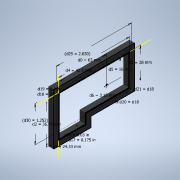
# Autodesk Inventor part: J010359
Saved by Autodesk Inventor 2020.3 (Build 243373000, 373)
## iProperties
RuleStatus: InUse
AfterDocSave0: file://Part Number Cleaner
Created: 2022-05-31
Part Number: J010359
Material: ACRYLIC, BLACK
Catalog Web Link: https://www.janelia.org/
Vendor: HHMI: JRC - jET
Document SubType Name: Modeling
Designer: arnoldj
Density: 1 g/cm^3
Appearance: Generic
Project: COMMON
Description: DOUT BASE PLATE
LAB/DEPT: COMMON
REQUESTING SCIENTIST: OCMMON
SURFACE ROUGHNESS: N/A
DESIGN DEPARTMENT: HHMI: JRC - jET
SPECIAL FINISH: NONE
ALTERED ITEM PART NUMBER: N/A
ALTERED ITEM VENDOR: N/A
ALTERED ITEM DESCRIPTION: N/A
Title: Standard
Author: arnoldj
Revision Number: 0
Autodesk Inventor part; units mm, degrees
ref_plane "YZ Plane" through (0, 0, 0) normal (1, 0, 0) x (0, 1, 0)
ref_plane "XZ Plane" through (0, 0, 0) normal (0, 1, 0) x (-1, 0, 0)
ref_plane "XY Plane" through (0, 0, 0) normal (0, 0, 1) x (1, 0, 0)
sketch "Sketch1" plane through (0, 0, 0) normal (1, 0, 0) x (0, 1, 0)
  line L0 (0, 18.823) -> (0, -81.823) projected
  line L1 (-50.323, 0) -> (13.573, 0) projected
  line L2 (0, 0) -> (0, -63)
  line L3 (0, -63) -> (-28, -63)
  line L4 (-28, -63) -> (-28, -24.33)
  line L5 (-28, -24.33) -> (-36.75, -24.33)
  line L6 (-36.75, -24.33) -> (-36.75, 0)
  line L7 (-36.75, 0) -> (0, 0)
  circle A0 centre (-16, -42.5) radius 1.575 construction
  line L8 (-35.988, -0.762) -> (-35.988, -23.568)
  line L9 (-35.988, -23.568) -> (-27.238, -23.568)
  line L10 (-27.238, -23.568) -> (-27.238, -62.238)
  line L11 (-27.238, -62.238) -> (-0.762, -62.238)
  line L12 (-0.762, -62.238) -> (-0.762, -0.762)
  line L13 (-0.762, -0.762) -> (-35.988, -0.762)
  line L14 (-41.195, 4.445) -> (-41.195, -28.775)
  line L15 (-41.195, -28.775) -> (-32.445, -28.775)
  line L16 (-32.445, -28.775) -> (-32.445, -67.445)
  line L17 (-32.445, -67.445) -> (4.445, -67.445)
  line L18 (4.445, -67.445) -> (4.445, 4.445)
  line L19 (4.445, 4.445) -> (-41.195, 4.445)
  line L20 (1.905, 1.905) -> (-29.905, 1.905) construction
  line L21 (-29.905, 1.905) -> (-29.905, -64.905) construction
  line L22 (-29.905, -64.905) -> (1.905, -64.905) construction
  line L23 (1.905, -64.905) -> (1.905, 1.905) construction
  dimension "d0" = 63
  dimension "d1" = 28
  dimension "d2" = 36.75
  dimension "d3" = 24.33
  dimension "d4" = 42.5
  dimension "d5" = 16
  dimension "d6" = 3.15
  dimension "d16" = 0.762
  dimension "d17" = 4.445
  dimension "d18" = 2.54
  dimension "d19" = 2.54
  dimension "d20" = 2.54
  dimension "d21" = 2.54
  dimension "d29" = 66.81
  dimension "d30" = 31.81
  constraints: 44 end point, 8 perpendicular, 3 horizontal, 2 coincident, 2 parallel, 2 point on line, 1 centre point, 10 other
  measures "d0" distance between parallel lines of L1 L3
  measures "d1" distance of L2.end L3.end
  measures "d2" distance between parallel lines of L6 L2
  measures "d3" distance of L5.end L6.end
  measures "d4" distance from line of L7 point (-16, -42.5)
  measures "d5" distance from line of point (-16, -42.5) L2
  measures "d6" diameter of A0
  measures "d16" distance between parallel lines of L6 L8
  measures "d17" distance between parallel lines of L6 L14
  measures "d18" distance between parallel lines of L23 L18
  measures "d19" distance between parallel lines of L20 L19
  measures "d20" distance between parallel lines of L21 L16
  measures "d21" distance between parallel lines of L22 L17
  measures "d29" distance of L22.end L20.start
  measures "d30" distance of L20.start L20.end
extrude "Extrusion1" add sketch "Sketch1" against normal blind 4.4958
hole "Hole1" at (0, -16, -42.5) direction (-1, 0, 0) diameter 3.15 end through all
hole "Hole2" at (0, 1.905, 1.905) at (0, -29.905, -64.905) direction (-1, 0, 0) diameter 2.6 end through all
equation "\"d20\" = d18"
equation "\"d21\" = d18"
body "Solid1"
